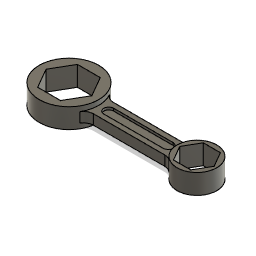
ex2 (Autodesk Fusion 360 design; units mm, degrees)
Autodesk Fusion 360 part; units mm, degrees
note: some values were not read from the file. Set by a fixed rule: which sketch regions a step uses.
sketch "Sketch1" plane through (0, 0, 0) normal (0, 1, 0) x (1, 0, 0)
  line L0 (0, 0) -> (129, 0)
  line L1 (11.547, -20) -> (23.094, 0)
  line L2 (23.094, 0) -> (11.547, 20)
  line L3 (11.547, 20) -> (-11.547, 20)
  line L4 (-11.547, 20) -> (-23.094, 0)
  line L5 (-23.094, 0) -> (-11.547, -20)
  line L6 (-11.547, -20) -> (11.547, -20)
  circle A0 centre (0, 0) radius 30
  circle A1 centre (129, 0) radius 20
  line L7 (129, 0) -> (129, -15)
  line L8 (137.6603, -15) -> (146.3205, 0)
  line L9 (146.3205, 0) -> (137.6603, 15)
  line L10 (137.6603, 15) -> (120.3397, 15)
  line L11 (120.3397, 15) -> (111.6795, 0)
  line L12 (111.6795, 0) -> (120.3397, -15)
  line L13 (120.3397, -15) -> (137.6603, -15)
  line L14 (45, 10) -> (111.6795, 10)
  line L15 (45, 10) -> (28.2843, 10)
  line L16 (45, -10) -> (28.2843, -10)
  line L17 (45, -10) -> (111.6795, -10)
  line L18 (40, -5) -> (109.6351, -5)
  line L19 (40, -5) -> (29.5804, -5)
  line L20 (40, 5) -> (109.6351, 5)
  line L21 (40, 5) -> (29.5804, 5)
  circle A2 centre (40, 0) radius 5
  circle A3 centre (100, 0) radius 5
  point P0 (129, 0)
  dimension "d1" = 129
  dimension "d3" = 60
  dimension "d4" = 40
  dimension "d5" = 15
  dimension "d9" = 20
  dimension "d10" = 10
  dimension "d11" = 10
  constraint coincident L0.start A0.centre
  constraint horizontal L0
  constraint coincident P0 L0.end
  constraint vertical L7
  constraint coincident A1 L14.end
  constraint coincident A0 L15.end
  constraint coincident A0 L16.end
  constraint coincident A1 L17.end
  constraint coincident A1 L18.end
  constraint coincident A0 L19.end
  constraint coincident A1 L20.end
  constraint coincident A0 L21.end
  constraint coincident L0 A2.centre
  constraint coincident L18.start A2
  constraint coincident L0 A3.centre
  constraint tangent L18 A3
  measures "d1" distance of L0.start P0
  measures "d3" diameter of A0
  measures "d4" diameter of A1
  measures "d5" distance of P0 L7.end
  measures "d9" distance of L14.start L16.start
  measures "d10" diameter of A2
  measures "d11" diameter of A3
extrude "Extrude1" add sketch "Sketch1" along normal mid plane 10 contours L0 A0 L21 A2 | L0 A0 L19 A2 | A0 A1 L14 L15 L20 L21 | A0 A1 L16 L17 L18 L19 | L0 A1 L20 A3 | L0 A1 L18 A3
extrude "Extrude2" add sketch "Sketch1" along normal mid plane 5 contours L0 A2 | L0 A2 | L0 L20 A2 A3 | L0 L18 A2 A3 | L0 A3 | L0 A3
extrude "Extrude3" add sketch "Sketch1" along normal mid plane 20 contours A0 | A1
fillet "Fillet1" radius 10 4 edges at (28.2843, 0, 10) (111.6795, 0, 10) (28.2843, 0, -10) (111.6795, 0, -10)
